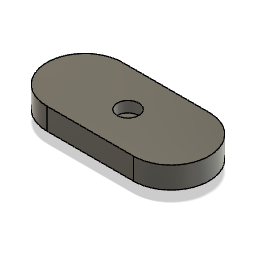
Base do meio v2 (Autodesk Fusion 360 design; units mm, degrees)
Autodesk Fusion 360 part; units mm, degrees
sketch "Sketch1" plane through (0, 0, 0) normal (0, 1, 0) x (1, 0, 0)
  line L0 (75, -35) -> (-75, -35)
  line L1 (-75, -35) -> (-75, 35)
  line L2 (-75, 35) -> (75, 35)
  line L3 (75, 35) -> (75, -35)
  line L4 (75, -35) -> (-75, 35) construction
  line L5 (-75, -35) -> (75, 35) construction
  dimension "d1" = 150
  dimension "d2" = 70
  constraint horizontal L0
  constraint perpendicular L0 L1
  constraint parallel L0 L2
  constraint parallel L1 L3
  constraint coincident L4 origin
  constraint coincident L5 origin
  measures "d1" distance of L1.end L2.end
  measures "d2" distance of L0.end L1.end
extrude "Extrude1" add sketch "Sketch1" along normal blind 20 makes body 1
fillet "Fillet1" radius 35 4 edges at (-75, 10, 35) (75, 10, 35) (75, 10, -35) (-75, 10, -35) on bodies 1
sketch "Sketch2" plane through (0, 0, 0) normal (0, -1, 0) x (1, 0, 0)
  arc A0 (-40, 35) -> (-40, -35) centre (-40, 0) ccw
  line L0 (-40, -35) -> (40, -35)
  arc A1 (40, -35) -> (40, 35) centre (40, 0) ccw
  line L1 (40, 35) -> (-40, 35)
  circle A2 centre (0, 0) radius 10
  dimension "d7" = 20
  constraint coincident A2.centre origin
  measures "d7" diameter of A2
extrude "Extrude2" add sketch "Sketch2" along normal blind 10 contours A2 bodies 1
sketch "Sketch3" plane through (0, 20, 0) normal (0, 1, 0) x (-1, 0, 0)
  arc A0 (40, -35) -> (40, 35) centre (40, 0) ccw
  line L0 (40, 35) -> (-40, 35)
  arc A1 (-40, 35) -> (-40, -35) centre (-40, 0) ccw
  line L1 (-40, -35) -> (40, -35)
  circle A2 centre (0, 0) radius 10
  dimension "d10" = 20
  constraint coincident A2.centre origin
  measures "d10" diameter of A2
extrude "Extrude3" cut sketch "Sketch3" against normal blind 10 contours A2 bodies 1
copy_body "Body->Comp1" bodies 1 removing the originals makes body 2 in component "Component"
component "Component" placed x (1, 0, 0) y (0, 1, 0) z (0, 0, 1) at (0, 0, 0)
